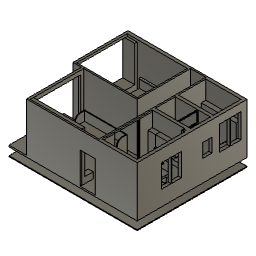
SmartHome-Model (Autodesk Fusion 360 design; units mm, degrees)
Autodesk Fusion 360 part; units mm, degrees
(part 1 of 2)
sketch "Frame" plane through (0, 0, 0) normal (0, 0, 1) x (1, 0, 0)
  line L0 (350, 350) -> (-350, 350)
  line L1 (-350, 350) -> (-350, -350)
  line L2 (-350, -350) -> (350, -350)
  line L3 (350, -350) -> (350, 350)
  line L4 (350, 350) -> (100, 350)
  line L5 (100, 350) -> (100, -350)
  line L6 (100, -350) -> (350, -350)
  line L7 (350, -350) -> (350, 350)
  line L8 (100, 350) -> (350, 350)
  line L9 (350, 350) -> (350, 150)
  line L10 (350, 150) -> (100, 150)
  line L11 (100, 150) -> (100, 350)
  line L12 (100, 150) -> (350, 150)
  line L13 (350, 150) -> (350, 0)
  line L14 (350, 0) -> (100, 0)
  line L15 (100, 0) -> (100, 150)
  line L16 (-350, 350) -> (0, 350)
  line L17 (0, 350) -> (0, 0)
  line L18 (0, 0) -> (-350, 0)
  line L19 (-350, 0) -> (-350, 350)
  line L20 (0, 350) -> (100, 350)
  line L21 (100, 350) -> (100, 280)
  line L22 (100, 280) -> (0, 280)
  line L23 (0, 280) -> (0, 350)
  line L24 (110, 340) -> (340, 340)
  line L25 (340, 340) -> (340, 160)
  line L26 (340, 160) -> (110, 160)
  line L27 (110, 160) -> (110, 340)
  line L28 (-360, 360) -> (-360, -360)
  line L29 (-360, -360) -> (360, -360)
  line L30 (360, -360) -> (360, 360)
  line L31 (360, 360) -> (-360, 360)
  line L32 (-10, 340) -> (-10, 10)
  line L33 (-10, 10) -> (-340, 10)
  line L34 (-340, 10) -> (-340, 340)
  line L35 (-10, 340) -> (-340, 340)
  line L36 (110, 140) -> (340, 140)
  line L37 (340, 140) -> (340, 10)
  line L38 (340, 10) -> (110, 10)
  line L39 (110, 10) -> (110, 140)
  line L40 (100, 0) -> (350, 0)
  line L41 (350, 0) -> (350, -350)
  line L42 (350, -350) -> (100, -350)
  line L43 (100, -350) -> (100, 0)
  line L44 (110, -10) -> (340, -10)
  line L45 (340, -10) -> (340, -340)
  line L46 (340, -340) -> (110, -340)
  line L47 (110, -340) -> (110, -10)
  line L48 (-360, -360) -> (-480, -360)
  line L49 (-480, -360) -> (-480, 0)
  line L50 (-480, 0) -> (-360, 0)
  line L51 (-360, 0) -> (-360, -360)
  dimension "d8" = 700
  dimension "d9" = 700
  dimension "d10" = 70
  dimension "d11" = 10
  dimension "d12" = 10
  dimension "d13" = -10
  dimension "d14" = 10
  dimension "d15" = 10
  dimension "d47" = 120
  constraint horizontal L0
  constraint perpendicular L0 L1
  constraint parallel L0 L2
  constraint parallel L1 L3
  constraint horizontal L4
  constraint vertical L5
  constraint horizontal L6
  constraint vertical L7
  constraint coincident L2 L5.end
  constraint horizontal L8
  constraint vertical L9
  constraint horizontal L10
  constraint vertical L11
  constraint coincident L7 L9.end
  constraint horizontal L12
  constraint vertical L13
  constraint horizontal L14
  constraint vertical L15
  constraint midpoint L7 L13.end
  constraint horizontal L16
  constraint vertical L17
  constraint horizontal L18
  constraint vertical L19
  constraint coincident L17.end L18.start
  constraint horizontal L20
  constraint vertical L21
  constraint horizontal L22
  constraint vertical L23
  constraint horizontal L40
  constraint vertical L41
  constraint horizontal L42
  constraint vertical L43
  constraint horizontal L48
  constraint vertical L49
  constraint horizontal L50
  constraint vertical L51
  measures "d8" distance of L1.end L2.end
  measures "d9" distance of L0.end L1.end
  measures "d10" distance of L16.end L22.end
  measures "d47" distance of L28.end L48.end
extrude "Extrude1" add sketch "Frame" along normal blind 320 contours L0 L3 L4 L5 L7 L8 L9 L10 L11 L12 L21 | L3 L5 L7 L10 L12 L13 L14 L15 L40 | L0 L1 L16 L17 L18 L19 L23 | L2 L3 L5 L6 L7 L14 L40 L41 L42 L43 | L28 L29 L30 L31 L51 makes body 1
sketch "Bedroom_Window" plane through (-340, 0, 0) normal (1, 0, 0) x (0, 1, 0)
  line L0 (10, 0) -> (340, 0)
  line L1 (340, 0) -> (340, 320)
  line L2 (340, 320) -> (10, 320)
  line L3 (10, 320) -> (10, 0)
  line L4 (10, 320) -> (340, 320)
  line L5 (340, 320) -> (340, 55)
  line L6 (340, 55) -> (10, 55)
  line L7 (10, 55) -> (10, 320)
  line L8 (25, 70) -> (25, 305)
  line L9 (25, 305) -> (325, 305)
  line L10 (325, 305) -> (325, 70)
  line L11 (325, 70) -> (25, 70)
  dimension "d20" = 265
  dimension "d21" = 15
  constraint horizontal L4
  constraint vertical L5
  constraint horizontal L6
  constraint vertical L7
  constraint coincident L2.end L3.start
  measures "d20" distance of L2.end L6.end
extrude "Extrude2" cut sketch "Bedroom_Window" against normal blind 20 contours L8 L9 L10 L11 bodies 1
extrude "Extrude3" add sketch "Frame" against normal blind 10 separate body contours L0 L3 L4 L5 L7 L8 L9 L10 L11 L12 L21 | L0 L5 L11 L17 L20 L21 L22 L23 | L3 L5 L7 L10 L12 L13 L14 L15 L40 | L0 L1 L16 L17 L18 L19 L23 | L1 L2 L5 L11 L15 L17 L18 L22 L43 | L2 L3 L5 L6 L7 L14 L40 L41 L42 L43 | L24 L25 L26 L27 | L28 L29 L30 L31 L51 | L32 L33 L34 L35 | L36 L37 L38 L39 | L44 L45 L46 L47 makes body 2
extrude "Extrude4" add sketch "Frame" along normal blind 120 contours L0 L5 L11 L17 L20 L21 L22 L23 bodies 1 2
sketch "Studyroom_Door" plane through (110, 0, 0) normal (1, 0, 0) x (0, 1, 0)
  line L0 (160, 0) -> (340, 0)
  line L1 (340, 0) -> (340, 320)
  line L2 (340, 320) -> (160, 320)
  line L3 (160, 320) -> (160, 0)
  line L4 (160, 0) -> (250, 0)
  line L5 (250, 0) -> (250, 200)
  line L6 (250, 200) -> (160, 200)
  line L7 (160, 200) -> (160, 0)
  dimension "d28" = 90
  dimension "d29" = 200
  constraint horizontal L4
  constraint vertical L5
  constraint horizontal L6
  constraint vertical L7
  constraint coincident L0.start L3.end
  measures "d28" distance of L0.start L4.end
  measures "d29" distance of L0.start L6.end
extrude "Extrude5" cut sketch "Studyroom_Door" against normal blind 10 contours L0 L3 L4 L5 L6 L7 bodies 1
extrude "Extrude6" cut sketch "Studyroom_Door" against normal blind 10 contours L0 L3 L4 L5 L6 L7 bodies 1
sketch "Frame_Maindoor" plane through (0, -350, 0) normal (0, 1, 0) x (-1, 0, 0)
  line L0 (-100, 0) -> (350, 0)
  line L1 (350, 0) -> (350, 320)
  line L2 (350, 320) -> (-100, 320)
  line L3 (-100, 320) -> (-100, 0)
  line L4 (-100, 0) -> (-85, 0)
  line L5 (-85, 0) -> (13, 0)
  line L6 (13, 0) -> (13, 206)
  line L7 (13, 206) -> (-85, 206)
  line L8 (-85, 206) -> (-85, 0)
  dimension "d34" = 15
  dimension "d35" = 98
  dimension "d36" = 206
  constraint coincident L0.start L3.end
  constraint perpendicular L3 L4
  constraint horizontal L5
  constraint vertical L6
  constraint horizontal L7
  constraint vertical L8
  measures "d34" distance of L0.start L4.end
  measures "d35" distance of L4.end L5.end
  measures "d36" distance of L4.end L7.end
extrude "Extrude7" cut sketch "Frame_Maindoor" against normal blind 20 contours L0 L5 L6 L7 L8 bodies 1
sketch "Bathroom_Door" plane through (110, 0, 0) normal (1, 0, 0) x (0, 1, 0)
  line L0 (140, 0) -> (50, 0)
  line L1 (50, 0) -> (50, 200)
  line L2 (50, 200) -> (140, 200)
  line L3 (140, 200) -> (140, 0)
  line L4 (140, 200) -> (130, 200)
  line L5 (130, 200) -> (130, 0)
  line L6 (130, 0) -> (140, 0)
  line L7 (140, 0) -> (140, 200)
  dimension "d39" = 90
  dimension "d40" = 200
  dimension "d41" = 10
  constraint horizontal L0
  constraint vertical L1
  constraint horizontal L2
  constraint vertical L3
  constraint horizontal L4
  constraint vertical L5
  constraint horizontal L6
  constraint vertical L7
  measures "d39" distance of L0.start L0.end
  measures "d40" distance of L0.start L2.end
  measures "d41" distance of L2.end L4.end
extrude "Extrude8" cut sketch "Bathroom_Door" against normal blind 10 contours L0 L1 L2 L5 bodies 1
sketch "Studyroom_Door_fix" plane through (0, 160, 0) normal (0, 1, 0) x (-1, 0, 0)
  line L0 (-340, 0) -> (-100, 0)
  line L1 (-100, 0) -> (-100, 200)
  line L2 (-100, 200) -> (-110, 200)
  line L3 (-110, 200) -> (-110, 320)
  line L4 (-110, 320) -> (-340, 320)
  line L5 (-340, 320) -> (-340, 0)
  line L6 (-100, 200) -> (-110, 200)
  line L7 (-110, 200) -> (-110, 0)
  line L8 (-110, 0) -> (-100, 0)
  line L9 (-100, 0) -> (-100, 200)
  constraint horizontal L6
  constraint vertical L7
  constraint horizontal L8
  constraint vertical L9
  constraint coincident L0 L7.end
  constraint coincident L1.end L2.start
extrude "Extrude9" add sketch "Studyroom_Door_fix" along normal blind 10 contours L0 L1 L2 L6 L7 L8 L9 bodies 1
move_face "OffsetFaces1" offset 60 1 faces at (-360, -231.6667, 126.6667) on bodies 1
extrude "Extrude10" add sketch "Frame" against normal blind 10 contours L28 L48 L49 L50 L51 bodies 1
sketch "Balcony_Door" plane through (0, 0, 320) normal (0, 0, 1) x (-1, 0, 0)
  line L0 (10, -340) -> (10, -10)
  line L1 (10, -10) -> (340, -10)
  line L2 (340, -10) -> (340, -340)
  line L3 (340, -340) -> (10, -340)
  line L4 (-340, 340) -> (-110, 340)
  line L5 (-110, 340) -> (-110, 10)
  line L6 (-110, 10) -> (-340, 10)
  line L7 (-340, 10) -> (-340, 340)
  line L8 (-340, -160) -> (-110, -160)
  line L9 (-110, -160) -> (-110, -340)
  line L10 (-110, -340) -> (-340, -340)
  line L11 (-340, -340) -> (-340, -160)
  line L12 (0, 0) -> (0, -350)
  line L13 (0, -350) -> (-100, -350)
  line L14 (-100, -350) -> (-100, 350)
  line L15 (-100, 350) -> (350, 350)
  line L16 (350, 350) -> (350, 0)
  line L17 (350, 0) -> (0, 0)
  line L18 (-340, -10) -> (-110, -10)
  line L19 (-110, -10) -> (-110, -140)
  line L20 (-110, -140) -> (-340, -140)
  line L21 (-340, -140) -> (-340, -10)
  line L22 (-360, -360) -> (420, -360)
  line L23 (420, -360) -> (420, 360)
  line L24 (420, 360) -> (-360, 360)
  line L25 (-360, 360) -> (-360, -360)
  line L26 (420, 350) -> (420, 330)
  line L27 (420, 0) -> (420, 20)
  line L28 (420, 330) -> (350, 330)
  line L29 (350, 330) -> (350, 20)
  line L30 (350, 20) -> (420, 20)
  line L31 (420, 20) -> (420, 330)
  constraint coincident L23 L26.start
  constraint coincident L23 L26.end
  constraint perpendicular L15 L26
  constraint coincident L23 L27.end
  constraint horizontal L28
  constraint vertical L29
  constraint horizontal L30
  constraint vertical L31
  constraint coincident L16 L29.end
extrude "Extrude11" cut sketch "Balcony_Door" against normal blind 320 contours L16 L23 L28 L29 L30 L31 bodies 1
sketch "Balcony_Door_fix1" plane through (0, 0, 320) normal (0, 0, 1) x (-1, 0, 0)
  line L0 (350, 330) -> (420, 330)
  line L1 (420, 330) -> (420, 360)
  line L2 (420, 360) -> (-360, 360)
  line L3 (-360, 360) -> (-360, -360)
  line L4 (-360, -360) -> (420, -360)
  line L5 (420, -360) -> (420, 20)
  line L6 (420, 20) -> (350, 20)
  line L7 (350, 20) -> (350, 0)
  line L8 (350, 0) -> (0, 0)
  line L9 (0, 0) -> (0, -350)
  line L10 (0, -350) -> (-100, -350)
  line L11 (-100, -350) -> (-100, 350)
  line L12 (-100, 350) -> (350, 350)
  line L13 (350, 350) -> (350, 330)
  line L14 (-340, -10) -> (-110, -10)
  line L15 (-110, -10) -> (-110, -140)
  line L16 (-110, -140) -> (-340, -140)
  line L17 (-340, -140) -> (-340, -10)
  line L18 (-340, -160) -> (-110, -160)
  line L19 (-110, -160) -> (-110, -340)
  line L20 (-110, -340) -> (-340, -340)
  line L21 (-340, -340) -> (-340, -160)
  line L22 (-340, 340) -> (-110, 340)
  line L23 (-110, 340) -> (-110, 10)
  line L24 (-110, 10) -> (-340, 10)
  line L25 (-340, 10) -> (-340, 340)
  line L26 (10, -340) -> (10, -10)
  line L27 (10, -10) -> (340, -10)
  line L28 (340, -10) -> (340, -340)
  line L29 (340, -340) -> (10, -340)
  line L30 (350, 0) -> (365, 0)
  line L31 (350, 350) -> (365, 350)
  line L32 (365, 350) -> (420, 350)
  line L33 (420, 350) -> (420, 0)
  line L34 (420, 0) -> (365, 0)
  line L35 (365, 0) -> (365, 350)
  dimension "d53" = 15
  dimension "d54" = 15
  dimension "d55" = 350
  constraint coincident L7.end L8.start
  constraint perpendicular L7 L30
  constraint coincident L12.end L13.start
  constraint perpendicular L13 L31
  constraint horizontal L32
  constraint vertical L33
  constraint horizontal L34
  constraint vertical L35
  measures "d53" distance of L7.end L30.end
  measures "d54" distance of L12.end L31.end
  measures "d55" distance of L31.end L30.end
extrude "Extrude12" cut sketch "Balcony_Door_fix1" against normal blind 320 contours L0 L1 L32 L33 L35 | L0 L6 L33 L35 | L5 L6 L33 L34 L35 bodies 1
move_face "OffsetFaces2" offset -55 1 faces at (-420, -353.3333, 213.3333) on bodies 1
sketch "Balcony_Door_fix2" plane through (0, 0, 320) normal (0, 0, 1) x (1, 0, 0)
  line L0 (-350, -20) -> (-365, -20)
  line L1 (-365, -20) -> (-365, -330)
  line L2 (-365, -330) -> (-350, -330)
  line L3 (-350, -330) -> (-350, -20)
  dimension "d59" = 15
  constraint horizontal L0
  constraint vertical L1
  constraint horizontal L2
  constraint vertical L3
  measures "d59" distance of L0.start L0.end
extrude "Extrude13" add sketch "Balcony_Door_fix2" against normal blind 25 bodies 1
sketch "Kitchen_Door_Frame" plane through (110, 0, 0) normal (1, 0, 0) x (0, 1, 0)
  line L0 (-340, 0) -> (-10, 0)
  line L1 (-10, 0) -> (-10, 320)
  line L2 (-10, 320) -> (-340, 320)
  line L3 (-340, 320) -> (-340, 0)
  line L4 (-340, 320) -> (-340, 310)
  line L5 (-340, 310) -> (-10, 310)
  line L6 (-10, 310) -> (-10, 5)
  line L7 (-10, 5) -> (-340, 5)
  line L8 (-340, 5) -> (-340, 310)
  dimension "d62" = 305
  constraint coincident L2.end L3.start
  constraint coincident L3 L4.end
  constraint perpendicular L2 L4
  constraint horizontal L5
  constraint vertical L6
  constraint horizontal L7
  constraint vertical L8
  measures "d62" distance of L4.end L7.end
extrude "Extrude14" cut sketch "Kitchen_Door_Frame" against normal blind 10 contours L1 L3 L5 L6 L7 L8 bodies 1
sketch "Bedroom_firniture" plane through (0, 0, 0) normal (0, 0, 1) x (-1, 0, 0)
  line L0 (10, -340) -> (340, -340)
  line L1 (340, -340) -> (340, -10)
  line L2 (340, -10) -> (10, -10)
  line L3 (10, -10) -> (10, -340)
  line L4 (10, -340) -> (76, -340)
  line L5 (76, -340) -> (76, -140)
  line L6 (76, -140) -> (10, -140)
  line L7 (10, -140) -> (10, -340)
  line L8 (81, -340) -> (131, -340)
  line L9 (131, -340) -> (131, -290)
  line L10 (131, -290) -> (81, -290)
  line L11 (81, -290) -> (81, -340)
  line L12 (131, -340) -> (136, -340)
  line L13 (136, -340) -> (316, -340)
  line L14 (316, -340) -> (316, -135)
  line L15 (316, -135) -> (136, -135)
  line L16 (136, -135) -> (136, -340)
  dimension "d65" = 66
  dimension "d66" = 200
  dimension "d67" = 5
  dimension "d68" = 50
  dimension "d69" = 50
  dimension "d70" = 5
  dimension "d71" = 180
  dimension "d72" = 205
  constraint horizontal L4
  constraint vertical L5
  constraint horizontal L6
  constraint vertical L7
  constraint coincident L0.start L3.end
  constraint horizontal L8
  constraint vertical L9
  constraint horizontal L10
  constraint vertical L11
  constraint perpendicular L9 L12
  constraint horizontal L13
  constraint vertical L14
  constraint horizontal L15
  constraint vertical L16
  measures "d65" distance of L0.start L4.end
  measures "d66" distance of L0.start L6.end
  measures "d67" distance of L4.end L8.start
  measures "d68" distance of L8.start L8.end
  measures "d69" distance of L8.start L10.end
  measures "d70" distance of L8.end L12.end
  measures "d71" distance of L12.end L13.end
  measures "d72" distance of L12.end L15.end
extrude "Extrude15" add sketch "Bedroom_firniture" along normal blind 220 separate body contours L0 L3 L4 L5 L6 L7 makes body 3
extrude "Extrude16" add sketch "Bedroom_firniture" along normal blind 50 separate body contours L0 L8 L9 L10 L11 makes body 4
extrude "Extrude17" add sketch "Bedroom_firniture" along normal blind 60 separate body contours L0 L13 L14 L15 L16 makes body 5
sketch "Bedroom_Bed_1" plane through (0, 0, 60) normal (0, 0, 1) x (-1, 0, 0)
  line L0 (136, -135) -> (136, -340)
  line L1 (136, -340) -> (316, -340)
  line L2 (316, -340) -> (316, -135)
  line L3 (316, -135) -> (136, -135)
  line L4 (316, -340) -> (136, -340)
  line L5 (136, -340) -> (136, -330)
  line L6 (136, -330) -> (316, -330)
  line L7 (316, -330) -> (316, -340)
  dimension "d79" = 10
  constraint horizontal L4
  constraint vertical L5
  constraint horizontal L6
  constraint vertical L7
  constraint coincident L1.end L2.start
  measures "d79" distance of L1.end L6.end
extrude "Extrude18" add sketch "Bedroom_Bed_1" along normal blind 60 contours L0 L1 L2 L4 L5 L6 L7 bodies 5
fillet "Fillet1" radius 2 1 edges at (-226, 340, 120) on bodies 5
fillet "Fillet2" radius 8 1 edges at (-226, 330, 120) on bodies 5
sketch "Frame_fix_bedroom_Baywindow" plane through (0, 0, 320) normal (0, 0, 1) x (-1, 0, 0)
  line L0 (350, 350) -> (350, 0)
  line L1 (350, 0) -> (0, 0)
  line L2 (0, 0) -> (0, -350)
  line L3 (0, -350) -> (-100, -350)
  line L4 (-100, -350) -> (-100, 350)
  line L5 (-100, 350) -> (350, 350)
  line L6 (365, 0) -> (365, 360)
  line L7 (365, 360) -> (-360, 360)
  line L8 (-360, 360) -> (-360, -360)
  line L9 (-360, -360) -> (420, -360)
  line L10 (420, -360) -> (420, 0)
  line L11 (420, 0) -> (365, 0)
  line L12 (-340, -10) -> (-110, -10)
  line L13 (-110, -10) -> (-110, -140)
  line L14 (-110, -140) -> (-340, -140)
  line L15 (-340, -140) -> (-340, -10)
  line L16 (-340, -160) -> (-110, -160)
  line L17 (-110, -160) -> (-110, -340)
  line L18 (-110, -340) -> (-340, -340)
  line L19 (-340, -340) -> (-340, -160)
  line L20 (-340, 340) -> (-110, 340)
  line L21 (-110, 340) -> (-110, 10)
  line L22 (-110, 10) -> (-340, 10)
  line L23 (-340, 10) -> (-340, 340)
  line L24 (10, -340) -> (10, -10)
  line L25 (10, -10) -> (340, -10)
  line L26 (340, -10) -> (340, -340)
  line L27 (340, -340) -> (10, -340)
  line L28 (340, -340) -> (405, -340)
  line L29 (405, -340) -> (405, -10)
  line L30 (405, -10) -> (340, -10)
  line L31 (340, -10) -> (340, -340)
  dimension "d86" = 65
  dimension "d87" = 330
  constraint horizontal L28
  constraint vertical L29
  constraint horizontal L30
  constraint vertical L31
  constraint coincident L26.end L27.start
  measures "d86" distance of L26.end L28.end
  measures "d87" distance of L26.end L25.end
extrude "Extrude19" cut sketch "Frame_fix_bedroom_Baywindow" against normal blind 15 contours L26 L28 L29 L30 L31 bodies 1
sketch "Bedroom_Door" plane through (-10, 0, 0) normal (-1, 0, 0) x (0, -1, 0)
  line L0 (-340, 0) -> (-10, 0)
  line L1 (-10, 0) -> (-10, 320)
  line L2 (-10, 320) -> (-340, 320)
  line L3 (-340, 320) -> (-340, 0)
  line L4 (-10, 0) -> (-20, 0)
  line L5 (-20, 0) -> (-100, 0)
  line L6 (-100, 0) -> (-100, 200)
  line L7 (-100, 200) -> (-20, 200)
  line L8 (-20, 200) -> (-20, 0)
  dimension "d90" = 10
  dimension "d91" = 80
  dimension "d92" = 200
  constraint coincident L0.end L1.start
  constraint perpendicular L1 L4
  constraint horizontal L5
  constraint vertical L6
  constraint horizontal L7
  constraint vertical L8
  measures "d90" distance of L0.end L4.end
  measures "d91" distance of L4.end L5.end
  measures "d92" distance of L4.end L7.end
extrude "Extrude20" cut sketch "Bedroom_Door" against normal blind 10 contours L0 L5 L6 L7 L8 bodies 1
sketch "Bathroom_Sketche" plane through (0, 0, 0) normal (0, 0, 1) x (-1, 0, 0)
  line L0 (365, 360) -> (365, 330)
  line L1 (365, 330) -> (350, 330)
  line L2 (350, 330) -> (350, 350)
  line L3 (350, 350) -> (13, 350)
  line L4 (13, 350) -> (13, 360)
  line L5 (13, 360) -> (-85, 360)
  line L6 (-85, 360) -> (-85, 350)
  line L7 (-85, 350) -> (-100, 350)
  line L8 (-100, 350) -> (-100, -50)
  line L9 (-100, -50) -> (-110, -50)
  line L10 (-110, -50) -> (-110, -10)
  line L11 (-110, -10) -> (-340, -10)
  line L12 (-340, -10) -> (-340, -140)
  line L13 (-340, -140) -> (-110, -140)
  line L14 (-110, -140) -> (-110, -130)
  line L15 (-110, -130) -> (-100, -130)
  line L16 (-100, -130) -> (-100, -170)
  line L17 (-100, -170) -> (-110, -170)
  line L18 (-110, -170) -> (-110, -160)
  line L19 (-110, -160) -> (-340, -160)
  line L20 (-340, -160) -> (-340, -340)
  line L21 (-340, -340) -> (-110, -340)
  line L22 (-110, -340) -> (-110, -250)
  line L23 (-110, -250) -> (-100, -250)
  line L24 (-100, -250) -> (-100, -280)
  line L25 (-100, -280) -> (0, -280)
  line L26 (0, -280) -> (0, -100)
  line L27 (0, -100) -> (10, -100)
  line L28 (10, -100) -> (10, -340)
  line L29 (10, -340) -> (340, -340)
  line L30 (340, -340) -> (340, -10)
  line L31 (340, -10) -> (10, -10)
  line L32 (10, -10) -> (10, -20)
  line L33 (10, -20) -> (0, -20)
  line L34 (0, -20) -> (0, 0)
  line L35 (0, 0) -> (350, 0)
  line L36 (350, 0) -> (350, 20)
  line L37 (350, 20) -> (365, 20)
  line L38 (365, 20) -> (365, 0)
  line L39 (365, 0) -> (420, 0)
  line L40 (420, 0) -> (480, 0)
  line L41 (480, 0) -> (480, 360)
  line L42 (480, 360) -> (365, 360)
  line L43 (-110, -50) -> (-182, -50)
  line L44 (-182, -50) -> (-182, -10)
  line L45 (-182, -10) -> (-110, -10)
  line L46 (-110, -10) -> (-110, -50)
  line L47 (-340, -140) -> (-260, -140)
  line L48 (-260, -140) -> (-260, -10)
  line L49 (-260, -10) -> (-340, -10)
  line L50 (-340, -10) -> (-340, -140)
  circle A0 centre (-220, -30) radius 20
  line L51 (-255, -140) -> (-255, -10)
  dimension "d95" = 72
  dimension "d96" = 5
  constraint horizontal L43
  constraint vertical L44
  constraint horizontal L45
  constraint vertical L46
  constraint coincident L9.end L10.start
  constraint horizontal L47
  constraint vertical L48
  constraint horizontal L49
  constraint vertical L50
  constraint coincident L11 L48.end
  constraint coincident L12.end L13.start
  measures "d95" distance of L9.end L43.end
extrude "Extrude21" add sketch "Bathroom_Sketche" along normal blind 320 contours L11 L13 L48 L51 bodies 1
sketch "Bathroom_washroom_Door" plane through (255, 0, 0) normal (-1, 0, 0) x (0, -1, 0)
  line L0 (-140, 0) -> (-10, 0)
  line L1 (-10, 0) -> (-10, 320)
  line L2 (-10, 320) -> (-140, 320)
  line L3 (-140, 320) -> (-140, 0)
  line L4 (-140, 320) -> (-10, 320)
  line L5 (-10, 320) -> (-10, 0)
  line L6 (-10, 0) -> (-140, 0)
  line L7 (-140, 0) -> (-140, 320)
  line L8 (-135, 315) -> (-15, 315)
  line L9 (-15, 315) -> (-15, 5)
  line L10 (-15, 5) -> (-135, 5)
  line L11 (-135, 5) -> (-135, 315)
  line L12 (-15, 250) -> (-135, 250)
  line L13 (-15, 245) -> (-135, 245)
  dimension "d99" = 5
  dimension "d100" = -5
  constraint horizontal L4
  constraint vertical L5
  constraint horizontal L6
  constraint vertical L7
  constraint coincident L0.end L1.start
  constraint coincident L2.end L3.start
  constraint coincident L11 L12.end
  constraint coincident L9 L12.start
extrude "Extrude22" cut sketch "Bathroom_washroom_Door" against normal blind 10 contours L8 L9 L11 L12 bodies 1
extrude "Extrude23" cut sketch "Bathroom_washroom_Door" against normal blind 10 contours L9 L10 L11 L13 bodies 1
move_face "OffsetFaces3" offset 50 1 faces at (256.6667, 15, 165) on bodies 1
sketch "Studyroom_Window" plane through (340, 0, 0) normal (-1, 0, 0) x (0, -1, 0)
  line L0 (-340, 0) -> (-160, 0)
  line L1 (-160, 0) -> (-160, 320)
  line L2 (-160, 320) -> (-340, 320)
  line L3 (-340, 320) -> (-340, 0)
  line L4 (-320, 110) -> (-180, 110)
  line L5 (-180, 110) -> (-180, 270)
  line L6 (-180, 270) -> (-320, 270)
  line L7 (-320, 270) -> (-320, 110)
  line L8 (-248, 110) -> (-248, 270)
  line L9 (-252, 110) -> (-252, 270)
  dimension "d106" = 140
  dimension "d107" = 160
  constraint horizontal L4
  constraint vertical L5
  constraint horizontal L6
  constraint vertical L7
  measures "d106" distance of L4.start L4.end
  measures "d107" distance of L4.start L6.end
extrude "Extrude24" cut sketch "Studyroom_Window" against normal blind 20 contours L4 L6 L7 L9 | L4 L5 L6 L8 bodies 1
sketch "Bathroom_Window" plane through (340, 0, 0) normal (-1, 0, 0) x (0, -1, 0)
  line L0 (-140, 0) -> (-10, 0)
  line L1 (-10, 0) -> (-10, 320)
  line L2 (-10, 320) -> (-140, 320)
  line L3 (-140, 320) -> (-140, 0)
  line L4 (-140, 0) -> (-130, 0)
  line L5 (-130, 0) -> (-130, 130)
  line L6 (-130, 130) -> (-70, 130)
  line L7 (-70, 130) -> (-70, 220)
  line L8 (-70, 220) -> (-130, 220)
  line L9 (-130, 220) -> (-130, 130)
  constraint coincident L0.start L3.end
  constraint coincident L0 L4.end
  constraint perpendicular L3 L4
  constraint perpendicular L4 L5
  constraint horizontal L6
  constraint vertical L7
  constraint horizontal L8
  constraint vertical L9
extrude "Extrude25" cut sketch "Bathroom_Window" against normal blind 20 contours L6 L7 L8 L9 bodies 1
sketch "Kitchen_Door_Slide" plane through (0, 0, 310) normal (0, 0, -1) x (1, 0, 0)
  line L0 (110, 10) -> (110, 340)
  line L1 (110, 340) -> (100, 340)
  line L2 (100, 340) -> (100, 10)
  line L3 (100, 10) -> (110, 10)
  line L4 (110, 10) -> (110, 92.5)
  line L5 (110, 340) -> (110, 257.5)
  line L6 (110, 10) -> (105, 10)
  line L7 (105, 10) -> (105, 92.5)
  line L8 (105, 92.5) -> (110, 92.5)
  line L9 (110, 92.5) -> (110, 10)
  line L10 (100, 10) -> (100, 15)
  line L11 (100, 15) -> (105, 15)
  line L12 (105, 15) -> (105, 97.5)
  line L13 (105, 97.5) -> (100, 97.5)
  line L14 (100, 97.5) -> (100, 15)
  line L15 (110, 257.5) -> (105, 257.5)
  line L16 (105, 257.5) -> (105, 340)
  line L17 (105, 340) -> (110, 340)
  line L18 (110, 340) -> (110, 257.5)
  line L19 (105, 340) -> (105, 335)
  line L20 (105, 335) -> (100, 335)
  line L21 (100, 335) -> (100, 252.5)
  line L22 (100, 252.5) -> (105, 252.5)
  line L23 (105, 252.5) -> (105, 335)
  dimension "d114" = 82.5
  dimension "d115" = 82.5
  dimension "d116" = 5
  dimension "d117" = 5
  dimension "d118" = 82.5
  dimension "d119" = 5
  dimension "d120" = 82.5
  constraint coincident L0.start L3.end
  constraint perpendicular L3 L4
  constraint coincident L0.end L1.start
  constraint perpendicular L1 L5
  constraint horizontal L6
  constraint vertical L7
  constraint horizontal L8
  constraint vertical L9
  constraint coincident L2.end L3.start
  constraint perpendicular L3 L10
  constraint horizontal L11
  constraint vertical L12
  constraint horizontal L13
  constraint vertical L14
  constraint horizontal L15
  constraint vertical L16
  constraint horizontal L17
  constraint vertical L18
  constraint coincident L16 L19.end
  constraint perpendicular L1 L19
  constraint horizontal L20
  constraint vertical L21
  constraint horizontal L22
  constraint vertical L23
  measures "d114" distance of L0.start L4.end
  measures "d115" distance of L0.end L5.end
  measures "d116" distance of L0.start L6.end
  measures "d117" distance of L2.end L10.end
  measures "d118" distance of L10.end L13.end
  measures "d119" distance of L5.end L15.end
  measures "d120" distance of L19.end L22.end
extrude "Extrude26" add sketch "Kitchen_Door_Slide" along normal blind 305 separate body contours L0 L3 L4 L6 L7 L8 L9 L12 | L0 L1 L5 L15 L16 L17 L18 L19 L23 | L2 L7 L11 L12 L13 L14 | L2 L16 L20 L21 L22 L23 makes body 6 at (110, -285, 208.3333) makes body 7 at (110, -37.5, 208.3333)
sketch "Kitchen_Sketche" plane through (0, 0, 0) normal (0, 0, 1) x (-1, 0, 0)
  line L0 (-340, 340) -> (-340, 10)
  line L1 (-340, 10) -> (-110, 10)
  line L2 (-110, 10) -> (-110, 340)
  line L3 (-110, 340) -> (-340, 340)
  line L4 (-110, 340) -> (-115, 340)
  line L5 (-115, 340) -> (-115, 335)
  line L6 (-115, 335) -> (-110, 335)
  line L7 (-110, 335) -> (-110, 340)
  line L8 (-115, 335) -> (-200, 335)
  line L9 (-200, 335) -> (-200, 265)
  line L10 (-200, 265) -> (-115, 265)
  line L11 (-115, 265) -> (-115, 335)
  line L12 (-110, 10) -> (-111, 10)
  line L13 (-280, 65) -> (-111, 65)
  line L14 (-111, 65) -> (-111, 10)
  line L15 (-340, 10) -> (-320, 10)
  line L16 (-320, 10) -> (-320, 30)
  line L17 (-320, 30) -> (-340, 30)
  line L18 (-340, 30) -> (-340, 10)
  line L19 (-340, 340) -> (-280, 340)
  line L20 (-280, 340) -> (-280, 65)
  circle A0 centre (-330, 20) radius 6
  circle A1 centre (-252.75, 37.5) radius 10
  circle A2 centre (-198.25, 37.5) radius 10
  line L21 (-280, 65) -> (-290, 65)
  line L22 (-290, 65) -> (-290, 10)
  line L23 (-290, 10) -> (-160, 10)
  line L24 (-111, 10) -> (-160, 10)
  line L25 (-160, 10) -> (-160, 40)
  line L26 (-160, 40) -> (-111, 40)
  line L27 (-111, 40) -> (-111, 10)
  dimension "d123" = 5
  dimension "d124" = 5
  dimension "d125" = 85
  dimension "d126" = 70
  dimension "d129" = 1
  dimension "d133" = 55
  dimension "d135" = 20
  dimension "d136" = 20
  dimension "d137" = 60
  dimension "d140" = 12
  dimension "d144" = 20
  dimension "d145" = 20
  dimension "d146" = 30
  constraint horizontal L4
  constraint vertical L5
  constraint horizontal L6
  constraint vertical L7
  constraint coincident L2.end L3.start
  constraint horizontal L8
  constraint vertical L9
  constraint horizontal L10
  constraint vertical L11
  constraint coincident L1.end L2.start
  constraint horizontal L12
  constraint horizontal L13
  constraint vertical L14
  constraint horizontal L15
  constraint vertical L16
  constraint horizontal L17
  constraint vertical L18
  constraint coincident L0.end L1.start
  constraint coincident L0.start L3.end
  constraint perpendicular L0 L19
  constraint perpendicular L20 L21
  constraint coincident L1 L22.end
  constraint perpendicular L1 L22
  constraint coincident L1 L23.end
  constraint horizontal L24
  constraint vertical L25
  constraint horizontal L26
  constraint vertical L27
  measures "d123" distance of L2.end L4.end
  measures "d124" distance of L2.end L6.end
  measures "d125" distance of L5.end L8.end
  measures "d126" distance of L5.end L10.end
  measures "d129" distance of L1.end L12.end
  measures "d133" distance of L12.end L13.end
  measures "d135" distance of L0.end L15.end
  measures "d136" distance of L0.end L17.end
  measures "d137" distance of L0.start L19.end
  measures "d140" diameter of A0
  measures "d144" diameter of A1
  measures "d145" diameter of A2
  measures "d146" distance of L12.end L26.end
extrude "Extrude27" add sketch "Kitchen_Sketche" along normal blind 185 separate body contours L8 L9 L10 L11 makes body 8
extrude "Extrude28" add sketch "Kitchen_Sketche" along normal blind 320 contours L0 L1 L15 L16 L17 L18 | A0 bodies 1
extrude "Extrude29" cut sketch "Kitchen_Sketche" along normal blind 320 contours A0 bodies 1
extrude "Extrude30" add sketch "Kitchen_Sketche" along normal blind 75 separate body contours L1 L13 L14 L21 L22 L23 L25 L26 makes body 9
extrude "Extrude31" add sketch "Kitchen_Sketche" along normal blind 75 contours L0 L1 L3 L16 L17 L19 L20 L21 L22 bodies 9
extrude "Extrude32" add sketch "Kitchen_Sketche" along normal blind 220 separate body contours L1 L14 L24 L25 L26 L27 makes body 10
extrude "Extrude33" add sketch "Kitchen_Sketche" along normal blind 74 contours A1 | A2 bodies 9
sketch "Kitchen_Cook_Holder" plane through (0, 0, 74) normal (0, 0, 1) x (-1, 0, 0)
  circle A0 centre (-198.25, 37.5) radius 10
  circle A1 centre (-198.25, 37.5) radius 9
  circle A2 centre (-198.25, 37.5) radius 8
  circle A3 centre (-198.25, 37.5) radius 7
  circle A4 centre (-198.25, 37.5) radius 6
  circle A5 centre (-198.25, 37.5) radius 5
  circle A6 centre (-198.25, 37.5) radius 4
  circle A7 centre (-198.25, 37.5) radius 3
  circle A8 centre (-198.25, 37.5) radius 2
  circle A9 centre (-198.25, 37.5) radius 1
  circle A10 centre (-252.75, 37.5) radius 9
  circle A11 centre (-252.75, 37.5) radius 10
  circle A12 centre (-252.75, 37.5) radius 8
  circle A13 centre (-252.75, 37.5) radius 7
  circle A14 centre (-252.75, 37.5) radius 6
  circle A15 centre (-252.75, 37.5) radius 5
  circle A16 centre (-252.75, 37.5) radius 4
  circle A17 centre (-252.75, 37.5) radius 3
  circle A18 centre (-252.75, 37.5) radius 2
  circle A19 centre (-252.75, 37.5) radius 1
  dimension "d155" = 18
  dimension "d156" = 16
  dimension "d157" = 14
  dimension "d158" = 12
  dimension "d159" = 10
  dimension "d160" = 8
  dimension "d161" = 6
  dimension "d162" = 4
  dimension "d163" = 2
  dimension "d164" = 18
  dimension "d165" = 16
  dimension "d166" = 14
  dimension "d167" = 12
  dimension "d168" = 10
  dimension "d169" = 8
  dimension "d170" = 6
  dimension "d171" = 4
  dimension "d172" = 2
  constraint concentric A0 A1
  constraint concentric A1 A2
  constraint concentric A2 A3
  constraint concentric A3 A4
  constraint concentric A4 A5
  constraint concentric A4 A6
  constraint concentric A5 A7
  constraint concentric A6 A8
  constraint concentric A4 A9
  constraint concentric A10 A11
  constraint concentric A11 A12
  constraint concentric A12 A13
  constraint concentric A12 A14
  constraint concentric A13 A15
  constraint concentric A13 A16
  constraint concentric A16 A17
  constraint concentric A14 A18
  constraint concentric A10 A19
  measures "d155" diameter of A1
  measures "d156" diameter of A2
  measures "d157" diameter of A3
  measures "d158" diameter of A4
  measures "d159" diameter of A5
  measures "d160" diameter of A6
  measures "d161" diameter of A7
  measures "d162" diameter of A8
  measures "d163" diameter of A9
  measures "d164" diameter of A10
  measures "d165" diameter of A12
  measures "d166" diameter of A13
  measures "d167" diameter of A14
  measures "d168" diameter of A15
  measures "d169" diameter of A16
  measures "d170" diameter of A17
  measures "d171" diameter of A18
  measures "d172" diameter of A19
extrude "Extrude34" add sketch "Kitchen_Cook_Holder" along normal blind 2 contours A1 | A3 | A5 | A7 | A9 | A10 | A13 | A15 | A17 | A19 bodies 9
sketch "Kitchen_Window" plane through (340, 0, 0) normal (-1, 0, 0) x (0, -1, 0)
  line L0 (30, 320) -> (30, 0)
  line L1 (30, 0) -> (340, 0)
  line L2 (340, 0) -> (340, 320)
  line L3 (340, 320) -> (30, 320)
  line L4 (30, 0) -> (340, 0)
  line L5 (340, 0) -> (340, 75)
  line L6 (340, 75) -> (30, 75)
  line L7 (30, 75) -> (30, 0)
  line L8 (70, 240) -> (200, 240)
  line L9 (200, 240) -> (200, 90)
  line L10 (200, 90) -> (70, 90)
  line L11 (70, 90) -> (70, 240)
  line L12 (133, 240) -> (133, 90)
  line L13 (137, 240) -> (137, 90)
  dimension "d175" = 75
  constraint horizontal L4
  constraint vertical L5
  constraint horizontal L6
  constraint vertical L7
  constraint coincident L0.end L1.start
  constraint horizontal L8
  constraint vertical L9
  constraint horizontal L10
  constraint vertical L11
  measures "d175" distance of L0.end L6.end
extrude "Extrude35" cut sketch "Kitchen_Window" against normal blind 20 contours L8 L9 L10 L13 bodies 1
extrude "Extrude36" cut sketch "Kitchen_Window" against normal blind 20 contours L8 L10 L11 L12 bodies 1
sketch "Kitchen_Furniture" plane through (0, 0, 75) normal (0, 0, 1) x (-1, 0, 0)
  circle A0 centre (-252.75, 37.5) radius 10
  circle A1 centre (-198.25, 37.5) radius 10
  line L0 (-111, 65) -> (-280, 65)
  line L1 (-280, 65) -> (-280, 340)
  line L2 (-280, 340) -> (-340, 340)
  line L3 (-340, 340) -> (-340, 30)
  line L4 (-340, 30) -> (-320, 30)
  line L5 (-320, 30) -> (-320, 10)
  line L6 (-320, 10) -> (-160, 10)
  line L7 (-160, 10) -> (-160, 40)
  line L8 (-160, 40) -> (-111, 40)
  line L9 (-111, 40) -> (-111, 65)
  line L10 (-340, 340) -> (-337, 340)
  line L11 (-337, 340) -> (-337, 335)
  line L12 (-337, 335) -> (-340, 335)
  line L13 (-340, 335) -> (-340, 340)
  line L14 (-337, 335) -> (-301, 335)
  line L15 (-301, 335) -> (-301, 289)
  line L16 (-301, 289) -> (-337, 289)
  line L17 (-337, 289) -> (-337, 335)
  line L18 (-280, 65) -> (-280, 100)
  line L19 (-330, 100) -> (-340, 100)
  line L20 (-330, 100) -> (-290, 100)
  line L21 (-290, 100) -> (-290, 180)
  line L22 (-290, 180) -> (-330, 180)
  line L23 (-330, 180) -> (-330, 100)
  line L24 (-330, 138.5) -> (-290, 138.5)
  line L25 (-330, 141.5) -> (-290, 141.5)
  line L26 (-337, 289) -> (-337, 284)
  line L27 (-337, 284) -> (-299, 284)
  line L28 (-299, 284) -> (-299, 232)
  line L29 (-299, 232) -> (-337, 232)
  line L30 (-337, 232) -> (-337, 284)
  line L31 (-337, 232) -> (-337, 225)
  line L32 (-337, 225) -> (-330, 225)
  line L33 (-330, 225) -> (-310, 225)
  line L34 (-310, 225) -> (-310, 188)
  line L35 (-310, 188) -> (-330, 188)
  line L36 (-330, 188) -> (-330, 225)
  dimension "d183" = 3
  dimension "d184" = 5
  dimension "d185" = 36
  dimension "d186" = 46
  dimension "d189" = 35
  dimension "d190" = 80
  dimension "d197" = 5
  dimension "d198" = 38
  dimension "d199" = 52
  dimension "d202" = 20
  dimension "d203" = 37
  constraint horizontal L10
  constraint vertical L11
  constraint horizontal L12
  constraint vertical L13
  constraint coincident L2.end L3.start
  constraint horizontal L14
  constraint vertical L15
  constraint horizontal L16
  constraint vertical L17
  constraint coincident L0.end L1.start
  constraint perpendicular L2 L18
  constraint coincident L3 L19.end
  constraint horizontal L20
  constraint vertical L21
  constraint horizontal L22
  constraint vertical L23
  constraint perpendicular L16 L26
  constraint horizontal L27
  constraint vertical L28
  constraint horizontal L29
  constraint vertical L30
  constraint perpendicular L29 L31
  constraint perpendicular L31 L32
  constraint horizontal L33
  constraint vertical L34
  constraint horizontal L35
  constraint vertical L36
  measures "d183" distance of L2.end L10.end
  measures "d184" distance of L2.end L12.end
  measures "d185" distance of L11.end L14.end
  measures "d186" distance of L11.end L16.end
  measures "d189" distance of L0.end L18.end
  measures "d190" distance of L19.start L22.end
  measures "d197" distance of L16.end L26.end
  measures "d198" distance of L26.end L27.end
  measures "d199" distance of L26.end L29.end
  measures "d202" distance of L32.end L33.end
  measures "d203" distance of L32.end L35.end
extrude "Extrude37" add sketch "Kitchen_Furniture" along normal blind 28 separate body contours L14 L15 L16 L17 makes body 11
extrude "Extrude38" cut sketch "Kitchen_Furniture" against normal blind 30 contours L20 L21 L23 L24 bodies 9
extrude "Extrude39" cut sketch "Kitchen_Furniture" against normal blind 30 contours L21 L22 L23 L25 bodies 9
extrude "Extrude40" add sketch "Kitchen_Furniture" along normal blind 32 separate body contours L27 L28 L29 L30 makes body 12
extrude "Extrude41" add sketch "Kitchen_Furniture" along normal blind 5 separate body contours L33 L34 L35 L36 makes body 13
sketch "Kitchen_washers" plane through (280, 0, 0) normal (-1, 0, 0) x (0, -1, 0)
  line L0 (65, 0) -> (340, 0)
  line L1 (340, 0) -> (340, 75)
  line L2 (340, 75) -> (65, 75)
  line L3 (65, 75) -> (65, 0)
  line L4 (340, 75) -> (180, 75)
  line L5 (180, 75) -> (180, 0)
  line L6 (180, 0) -> (340, 0)
  line L7 (340, 0) -> (340, 75)
  line L8 (180, 75) -> (190, 75)
  line L9 (190, 75) -> (190, 65)
  line L10 (190, 65) -> (180, 65)
  line L11 (180, 65) -> (180, 75)
  line L12 (340, 75) -> (330, 75)
  line L13 (330, 75) -> (330, 65)
  line L14 (330, 65) -> (340, 65)
  line L15 (340, 65) -> (340, 75)
  line L16 (330, 65) -> (265, 65)
  line L17 (265, 65) -> (265, 0)
  line L18 (265, 0) -> (330, 0)
  line L19 (330, 0) -> (330, 65)
  line L20 (190, 65) -> (255, 65)
  line L21 (255, 65) -> (255, 0)
  line L22 (255, 0) -> (190, 0)
  line L23 (190, 0) -> (190, 65)
  line L24 (191, 0) -> (191, 64)
  line L25 (191, 64) -> (254, 64)
  line L26 (254, 64) -> (254, 0)
  line L27 (329, 0) -> (329, 64)
  line L28 (329, 64) -> (266, 64)
  line L29 (266, 64) -> (266, 0)
  dimension "d206" = 160
  dimension "d207" = 10
  dimension "d208" = 10
  dimension "d210" = 65
  dimension "d215" = 1
  dimension "d216" = -1
  constraint horizontal L4
  constraint vertical L5
  constraint horizontal L6
  constraint vertical L7
  constraint coincident L1.end L2.start
  constraint horizontal L8
  constraint vertical L9
  constraint horizontal L10
  constraint vertical L11
  constraint horizontal L12
  constraint vertical L13
  constraint horizontal L14
  constraint vertical L15
  constraint horizontal L16
  constraint vertical L17
  constraint horizontal L18
  constraint vertical L19
  constraint horizontal L20
  constraint vertical L21
  constraint horizontal L22
  constraint vertical L23
  constraint coincident L0 L21.end
  constraint coincident L6 L21.end
  measures "d206" distance of L1.end L4.end
  measures "d207" distance of L4.end L8.end
  measures "d208" distance of L4.end L10.end
  measures "d210" distance of L13.end L16.end
extrude "Extrude42" cut sketch "Kitchen_washers" against normal blind 60 contours L0 L6 L20 L21 L22 L23 L24 L25 L26 | L0 L6 L22 L24 L25 L26 bodies 9
extrude "Extrude43" cut sketch "Kitchen_washers" against normal blind 60 contours L0 L6 L16 L17 L18 L19 L27 L28 L29 | L0 L6 L18 L27 L28 L29 bodies 9
extrude "Extrude44" add sketch "Kitchen_washers" against normal blind 59 separate body contours L0 L6 L22 L24 L25 L26 makes body 14
extrude "Extrude45" add sketch "Kitchen_washers" against normal blind 59 separate body contours L0 L6 L18 L27 L28 L29 makes body 15
sketch "Holder" plane through (0, 0, -10) normal (0, 0, -1) x (1, 0, 0)
  line L0 (-420, 0) -> (-420, -360)
  line L1 (-420, -360) -> (360, -360)
  line L2 (360, -360) -> (360, 360)
  line L3 (360, 360) -> (-480, 360)
  line L4 (-480, 360) -> (-480, 0)
  line L5 (-480, 0) -> (-420, 0)
  line L6 (360, -360) -> (-480, -360)
  line L7 (-480, -360) -> (-480, 360)
  line L8 (-480, 360) -> (360, 360)
  line L9 (360, 360) -> (360, -360)
  constraint horizontal L6
  constraint vertical L7
  constraint horizontal L8
  constraint vertical L9
  constraint coincident L3.end L4.start
  constraint coincident L1.end L2.start
extrude "Extrude46" add sketch "Holder" along normal blind 55 separate body makes body 16
move_face "OffsetFaces4" offset -50 1 faces at (80, 0, -10) on bodies 16
sketch "Kitchen_range_hood" plane through (0, -10, 0) normal (0, -1, 0) x (1, 0, 0)
  line L0 (320, 0) -> (320, 320)
  line L1 (320, 320) -> (110, 320)
  line L2 (110, 320) -> (110, 310)
  line L3 (110, 310) -> (100, 310)
  line L4 (100, 310) -> (100, 5)
  line L5 (100, 5) -> (110, 5)
  line L6 (110, 5) -> (110, 0)
  line L7 (110, 0) -> (320, 0)
  line L8 (160, 75) -> (290, 75)
  line L9 (290, 75) -> (290, 220)
  line L10 (290, 220) -> (160, 220)
  line L11 (160, 220) -> (160, 75)
  line L12 (160, 75) -> (160, 105)
  line L13 (160, 105) -> (290, 105)
  line L14 (290, 105) -> (290, 140)
  line L15 (290, 140) -> (160, 140)
  line L16 (160, 140) -> (160, 105)
  line L17 (160, 150) -> (290, 150)
  line L18 (290, 150) -> (290, 140)
  line L19 (290, 140) -> (160, 140)
  line L20 (160, 140) -> (160, 150)
  line L21 (160, 150) -> (290, 150)
  line L22 (290, 150) -> (290, 153)
  line L23 (290, 153) -> (160, 153)
  line L24 (160, 153) -> (160, 150)
  line L25 (160, 153) -> (290, 153)
  line L26 (290, 153) -> (290, 220)
  line L27 (290, 220) -> (160, 220)
  line L28 (160, 220) -> (160, 153)
  dimension "d224" = 130
  dimension "d225" = 145
  dimension "d226" = 30
  dimension "d231" = 3
  constraint horizontal L8
  constraint vertical L9
  constraint horizontal L10
  constraint vertical L11
  constraint perpendicular L8 L12
  constraint horizontal L13
  constraint vertical L14
  constraint horizontal L15
  constraint vertical L16
  constraint coincident L9 L14.end
  constraint horizontal L17
  constraint vertical L18
  constraint horizontal L19
  constraint vertical L20
  constraint coincident L11 L17.start
  constraint horizontal L21
  constraint vertical L22
  constraint horizontal L23
  constraint vertical L24
  constraint horizontal L25
  constraint vertical L26
  constraint horizontal L27
  constraint vertical L28
  measures "d224" distance of L8.start L8.end
  measures "d225" distance of L8.start L10.end
  measures "d226" distance of L8.start L12.end
  measures "d231" distance of L17.start L23.end
extrude "Extrude47" add sketch "Kitchen_range_hood" along normal blind 40 separate body contours L9 L11 L13 L14 L15 L16 L19 | L9 L11 L15 L17 L18 L19 L20 L21 makes body 17
extrude "Extrude48" add sketch "Kitchen_range_hood" along normal blind 30 separate body contours L9 L10 L11 L23 L25 L26 L27 L28 makes body 18
draft "Draft2" angle -45 neutral plane through (0, -10, 0) pull (0, 1, 0) 1 faces at (203.3333, -23.3333, 105) on bodies 17
sketch "Studyroom_Sketche" plane through (0, 0, 0) normal (0, 0, 1) x (-1, 0, 0)
  line L0 (-255, -10) -> (-255, -140)
  line L1 (-255, -140) -> (-110, -140)
  line L2 (-110, -140) -> (-110, -130)
  line L3 (-110, -130) -> (-100, -130)
  line L4 (-100, -130) -> (-100, -170)
  line L5 (-100, -170) -> (-110, -170)
  line L6 (-110, -170) -> (-110, -160)
  line L7 (-110, -160) -> (-340, -160)
  line L8 (-340, -160) -> (-340, -340)
  line L9 (-340, -340) -> (-110, -340)
  line L10 (-110, -340) -> (-110, -250)
  line L11 (-110, -250) -> (-100, -250)
  line L12 (-100, -250) -> (-100, -280)
  line L13 (-100, -280) -> (0, -280)
  line L14 (0, -280) -> (0, -100)
  line L15 (0, -100) -> (10, -100)
  line L16 (10, -100) -> (10, -340)
  line L17 (10, -340) -> (340, -340)
  line L18 (340, -340) -> (340, -10)
  line L19 (340, -10) -> (10, -10)
  line L20 (10, -10) -> (10, -20)
  line L21 (10, -20) -> (0, -20)
  line L22 (0, -20) -> (0, 0)
  line L23 (0, 0) -> (350, 0)
  line L24 (350, 0) -> (350, 20)
  line L25 (350, 20) -> (365, 20)
  line L26 (365, 20) -> (365, 0)
  line L27 (365, 0) -> (420, 0)
  line L28 (420, 0) -> (480, 0)
  line L29 (480, 0) -> (480, 360)
  line L30 (480, 360) -> (365, 360)
  line L31 (365, 360) -> (365, 330)
  line L32 (365, 330) -> (350, 330)
  line L33 (350, 330) -> (350, 350)
  line L34 (350, 350) -> (13, 350)
  line L35 (13, 350) -> (13, 360)
  line L36 (13, 360) -> (-85, 360)
  line L37 (-85, 360) -> (-85, 350)
  line L38 (-85, 350) -> (-100, 350)
  line L39 (-100, 350) -> (-100, -50)
  line L40 (-100, -50) -> (-110, -50)
  line L41 (-110, -50) -> (-110, -10)
  line L42 (-110, -10) -> (-255, -10)
  line L43 (-340, -340) -> (-110, -340)
  line L44 (-110, -340) -> (-110, -310)
  line L45 (-110, -310) -> (-340, -310)
  line L46 (-340, -310) -> (-340, -340)
  line L47 (-340, -310) -> (-280, -310)
  line L48 (-280, -310) -> (-280, -160)
  line L49 (-280, -160) -> (-340, -160)
  line L50 (-340, -160) -> (-340, -310)
  circle A0 centre (-330, -300) radius 4
  circle A1 centre (-290, -300) radius 4
  circle A2 centre (-330, -170) radius 4
  circle A3 centre (-290, -170) radius 4
  dimension "d236" = 8
  dimension "d237" = 8
  dimension "d238" = 8
  dimension "d239" = 8
  constraint horizontal L43
  constraint vertical L44
  constraint horizontal L45
  constraint vertical L46
  constraint coincident L10 L44.end
  constraint coincident L8.end L9.start
  constraint horizontal L47
  constraint vertical L48
  constraint horizontal L49
  constraint vertical L50
  constraint coincident L7 L48.end
  measures "d236" diameter of A0
  measures "d237" diameter of A1
  measures "d238" diameter of A2
  measures "d239" diameter of A3
extrude "Extrude49" add sketch "Studyroom_Sketche" along normal blind 72 separate body contours L7 L8 L45 L47 L48 L49 L50 | A0 | A1 | A2 | A3 makes body 19
extrude "Extrude50" cut sketch "Studyroom_Sketche" along normal blind 70 contours L7 L8 L45 L47 L48 L49 L50 bodies 19
extrude "Extrude51" add sketch "Studyroom_Sketche" along normal blind 200 contours L8 L9 L10 L43 L44 L45 L46 L47 bodies 19